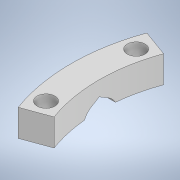
# Autodesk Inventor part: cable_jig_clamp
Saved by Autodesk Inventor 2022 (Build 260153000, 153)
## iProperties
Created: 2022-03-09
Part Number: cable_jig_clamp
Material: Generic
Document SubType Name: Modeling
Designer: kylem
Density: 1 g/cm^3
Appearance: Default
Author: kylem
Autodesk Inventor part; units mm, degrees
ref_plane "YZ Plane" through (0, 0, 0) normal (1, 0, 0) x (0, 1, 0)
ref_plane "XZ Plane" through (0, 0, 0) normal (0, 1, 0) x (-1, 0, 0)
ref_plane "XY Plane" through (0, 0, 0) normal (0, 0, 1) x (1, 0, 0)
sketch "Sketch1" plane through (0, 0, 0) normal (0, 1, 0) x (-1, 0, 0)
  circle A0 centre (0, 0) radius 34.95
  circle A1 centre (0, 0) radius 29.75
  line L0 (0, 0) -> (41.2193, -15.0026)
  line L1 (0, 0) -> (43.8647, 0) construction
  line L2 (0, 0) -> (47.0412, -17.1216)
  line L3 (0, 0) -> (50.0602, 0) construction
  line L4 (0, 0) -> (41.5964, 15.1399)
  line L5 (0, 0) -> (44.266, 0) construction
  point P0 (32.8423, 11.9536)
  point P1 (27.9559, 10.1751)
  point P2 (27.9559, -10.1751)
  point P3 (32.8423, -11.9536)
  dimension "d0" = 69.9
  dimension "d1" = 59.5
  dimension "d2" = 20
  dimension "d3" = 340
  dimension "d4" = 20
  constraints: 12 end point, 3 equal length, 3 horizontal, 2 centre point, 2 coincident
  measures "d0" diameter of A0
  measures "d1" diameter of A1
  measures "d2" angle of L0 L1
  measures "d4" angle of L5 L4
extrude "Extrusion1" add sketch "Sketch1" along normal blind 5 contours A0 L0 A1 L4 picked at (33.1379, 1.3525)
sketch "Sketch2" plane through (0, 0, 0) normal (1, 0, 0) x (0, 1, 0)
  line L0 (0, 0) -> (0, -1)
  line L1 (0, 10.1751) -> (0, -10.1751) projected
  line L2 (0, -1) -> (0, 1)
  line L3 (0, 0) -> (1, 0)
  line L4 (1, 0) -> (0, 1)
  line L5 (0, 0) -> (-1.5, 0)
  circle A0 centre (-1.5, 0) radius 3.25
  line L6 (1.75, 0) -> (2.25, 0)
  line L7 (2.25, 0) -> (1.3167, -1.6214)
  line L8 (2.25, 0) -> (1.3167, 1.6214)
  point P0 (0, 2.8831)
  point P1 (0, -2.8831)
  dimension "d7" = 1
  dimension "d8" = 2
  dimension "d9" = 1
  dimension "d16" = 1.5
  dimension "d17" = 6.5
  dimension "d18" = 0.5
  constraints: 16 end point, 3 point on circle, 2 perpendicular, 2 point on line, 2 tangent, 1 centre point, 1 coincident, 1 horizontal
  measures "d7" distance of L0.start L0.end
  measures "d8" distance of L0.end L2.end
  measures "d9" distance of L0.start L3.end
  measures "d16" distance of L0.start L5.end
  measures "d17" diameter of A0
  measures "d18" distance of L6.start L6.end
sketch "Sketch3" plane through (0, 5, 0) normal (0, 1, 0) x (1, 0, 0)
  line L0 (0, 0) -> (-39.1232, 10.483)
  line L1 (0, 0) -> (40.5033, 0) construction
  line L2 (0, 0) -> (-4.9273, 0)
  arc A0 (-32.8423, 11.9536) -> (-32.8423, -11.9536) centre (0, 0) ccw projected
  line L3 (-33.7591, 9.0457) -> (-28.7363, 7.6999)
  arc A1 (-27.9559, 10.1751) -> (-27.9559, -10.1751) centre (0, 0) ccw projected
  circle A2 centre (-31.2477, 8.3728) radius 1.65
  circle A3 centre (-31.2477, -8.3728) radius 1.65
  dimension "d12" = 165
  dimension "d13" = 3.3
  constraints: 8 end point, 2 centre point, 2 horizontal, 2 point on circle, 2 point on line, 1 equal length, 1 midpoint, 1 symmetric about line, 1 other
  measures "d12" angle of L1 L0
  measures "d13" diameter of A2
extrude "Extrusion3" cut sketch "Sketch3" against normal blind 100
extrude "Extrusion4" cut sketch "Sketch2" against normal blind 200 contours L3 L4 L1 A0 L0 | L1 L4 L3 | A0 L6 L7 | L8 L6 A0
body "Solid1"
